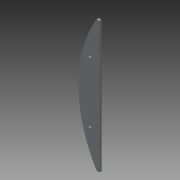
# Autodesk Inventor part: naraznik_kryt
Saved by Autodesk Inventor 2015 (Build 190159000, 159)
## iProperties
Created: 2015-01-01
Part Number: naraznik_kryt
Material: Generic
Document SubType Name: Modeling
Designer: Turboslimak
Density: 1 g/cm^3
Appearance: Default
Author: Turboslimak
Autodesk Inventor part; units mm, degrees
ref_plane "YZ Plane" through (0, 0, 0) normal (1, 0, 0) x (0, 1, 0)
ref_plane "XZ Plane" through (0, 0, 0) normal (0, 1, 0) x (-1, 0, 0)
ref_plane "XY Plane" through (0, 0, 0) normal (0, 0, 1) x (1, 0, 0)
sketch "Sketch1" plane through (0, 0, 0) normal (0, 1, 0) x (-1, 0, 0)
  line L0 (-10.5, 65.5) -> (-10.5, -65.5)
  line L1 (-10.5, 65.5) -> (-7.5, 65.5)
  line L2 (-10.5, -65.5) -> (-7.5, -65.5)
  arc A0 (-7.5, -65.5) -> (-7.5, 65.5) centre (-117.6736, 0) ccw
  line L3 (-7.5, 65.5) -> (-10.5, 65.5)
  line L4 (-10.5, 65.5) -> (-10.5, -65.5)
  line L5 (-10.5, -65.5) -> (-7.5, -65.5)
  line L6 (-10.5, -65.5) -> (-10.5, 65.5)
  line L7 (-10.5, -65.5) -> (-10.5, -30.5)
  line L8 (-10.5, 65.5) -> (-10.5, 30.15)
  line L9 (-10.5, 30.5) -> (-10.5, -30.5)
  line L10 (-10.5, 30.5) -> (-10.5, -30.5)
  circle A1 centre (-0.5, -30.5) radius 1.5
  line L11 (-0.5, -30.5) -> (-10.5, -30.5)
  line L12 (-10.5, -30.5) -> (-10.5, 30.15)
  line L13 (-10.5, 30.15) -> (-0.5, 30.15)
  circle A2 centre (-0.5, 30.15) radius 1.5
  point P0 (0, 0)
  dimension "d2" = 3
  dimension "d3" = 3
  dimension "d13" = 35
  dimension "d14" = 35.35
  dimension "d17" = 3
  dimension "d21" = 3
  constraints: 28 end point, 3 centre point, 3 perpendicular, 2 horizontal, 2 point on circle, 2 point on line, 1 coincident, 1 parallel
  measures "d2" distance of L0.start L1.end
  measures "d3" distance of L0.end L2.end
  measures "d13" distance of L6.start L7.end
  measures "d14" distance of L0.start L8.end
  measures "d17" diameter of A1
  measures "d21" diameter of A2
extrude "Extrusion1" add sketch "Sketch1" along normal blind 2 contours A2 | A1 | L1 A0 L2 L0
extrude "Extrusion3" cut sketch "Sketch1" along normal blind 2 contours A2 | A1
body "Solid1"
